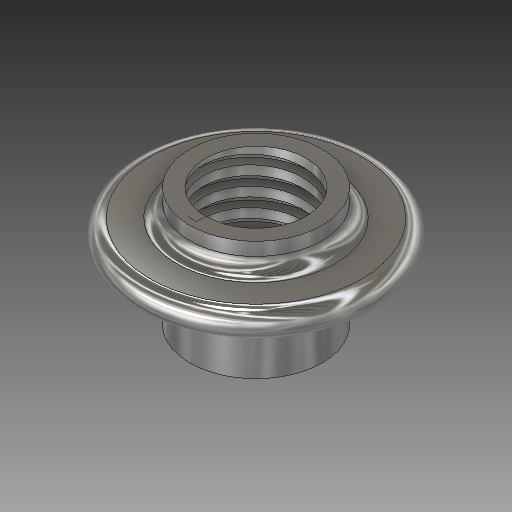
# Autodesk Inventor part: Nut
Saved by Autodesk Inventor 2018 (Build 220112000, 112)
## iProperties
Created: 2019-08-28
Part Number: Nut
Material: Generic
Document SubType Name: Modeling
Designer: HP
Density: 1 g/cm^3
Appearance: Chrome - Polished
Author: HP
Autodesk Inventor part; units mm, degrees
ref_plane "YZ Plane" through (0, 0, 0) normal (1, 0, 0) x (0, 1, 0)
ref_plane "XZ Plane" through (0, 0, 0) normal (0, 1, 0) x (-1, 0, 0)
ref_plane "XY Plane" through (0, 0, 0) normal (0, 0, 1) x (1, 0, 0)
sketch "Sketch1" plane through (0, 0, 0) normal (0, 0, 1) x (1, 0, 0)
  line L0 (25, 0) -> (19, 0)
  line L1 (19, 0) -> (19, 45)
  line L2 (19, 45) -> (25, 45)
  line L3 (25, 45) -> (25, 40)
  line L4 (30, 35) -> (40, 35)
  line L5 (40, 25) -> (25, 25)
  line L6 (25, 25) -> (25, 0)
  arc A0 (40, 25) -> (40, 35) centre (40, 30) ccw
  arc A1 (25, 40) -> (30, 35) centre (30, 40) ccw
  line L7 (0, -9) -> (0, 54) projected
  point P0 (0, 0)
  constraints: 14 end point, 4 perpendicular, 4 point on circle, 2 centre point, 1 horizontal, 1 point on line
revolve "Revolution1" add sketch "Sketch1" angle 360 about axis through (0, -10, 0) along (0, 1, 0)
sketch "Sketch2" plane through (0, 0, 0) normal (1, 0, 0) x (0, 1, 0)
  line L0 (45, 19) -> (45, -19) projected
  line L1 (45, 19) -> (41.5, 19)
  line L2 (41.5, 22.5) -> (45, 22.5)
  line L3 (45, 22.5) -> (45, 19)
  line L4 (45, 19) -> (41.5, 19)
  line L5 (41.5, 19) -> (41.5, 22.5)
  point P0 (0, 0)
  dimension "d15" = 3.5
  constraints: 10 end point, 2 perpendicular, 1 horizontal
  measures "d15" distance of L0.start L1.end
coil "Coil1" sketch "Sketch2" operation cut axis through (0, -10, 0) along (0, -1, 0) pitch 7 turns 8 hand right
body "Solid1"
